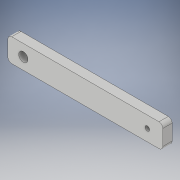
# Autodesk Inventor part: Fourbar-Crank
Saved by Autodesk Inventor 2019 (Build 230136000, 136)
## iProperties
Created: 2021-06-06
Part Number: Fourbar-Crank
Material: Generic
Document SubType Name: Modeling
Designer: micha
Density: 1 g/cm^3
Appearance: Default
Author: micha
Autodesk Inventor part; units mm, degrees
ref_plane "YZ Plane" through (0, 0, 0) normal (1, 0, 0) x (0, 1, 0)
ref_plane "XZ Plane" through (0, 0, 0) normal (0, 1, 0) x (-1, 0, 0)
ref_plane "XY Plane" through (0, 0, 0) normal (0, 0, 1) x (1, 0, 0)
sketch "Sketch1" plane through (0, 0, 0) normal (0, 0, 1) x (1, 0, 0)
  line L0 (0, 0) -> (200, 0)
  line L1 (200, 0) -> (200, 30)
  line L2 (200, 30) -> (0, 30)
  line L3 (0, 30) -> (0, 0)
  dimension "d0" = 200
  dimension "d1" = 30
  constraints: 8 end point, 2 parallel, 1 horizontal, 1 perpendicular
  measures "d0" distance of L2.end L1.end
  measures "d1" distance of L1.end L0.end
extrude "Extrusion1" add sketch "Sketch1" along normal blind 12
fillet "Fillet1" radius 5 4 edges at (200, 30, 6) (200, 0, 6) (0, 0, 6) (0, 30, 6)
sketch "Sketch2" plane through (0, 0, 12) normal (0, 0, 1) x (1, 0, 0)
  line L0 (0, 25) -> (0, 5) projected
  line L1 (0, 15) -> (20, 15)
  circle A0 centre (20, 15) radius 6
  line L2 (5, 0) -> (195, 0) projected
  line L3 (100, 0) -> (100, 30)
  line L4 (195, 30) -> (5, 30) projected
  line L5 (200, 5) -> (200, 25) projected
  line L6 (200, 15) -> (180, 15)
  circle A1 centre (180, 15) radius 3
  point P0 (0, 0)
  dimension "d5" = 20
  dimension "d6" = 12
  dimension "d10" = 20
  dimension "d11" = 6
  constraints: 6 end point, 4 midpoint, 2 centre point, 2 coincident, 1 horizontal, 1 parallel
  measures "d5" distance of L1.start L1.end
  measures "d6" diameter of A0
  measures "d10" distance of L6.start L6.end
  measures "d11" diameter of A1
extrude "Extrusion2" cut sketch "Sketch2" against normal through all
body "Solid1"
